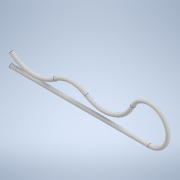
# Autodesk Inventor part: Pin
Saved by Autodesk Inventor 2022 (Build 260153000, 153)
## iProperties
Created: 2022-04-12
Part Number: Pin
Material: Generic
Document SubType Name: Modeling
Designer: Patrick
Density: 1 g/cm^3
Appearance: Default
Author: Patrick
Autodesk Inventor part; units mm, degrees
ref_plane "YZ Plane" through (0, 0, 0) normal (1, 0, 0) x (0, 1, 0)
ref_plane "XZ Plane" through (0, 0, 0) normal (0, 1, 0) x (-1, 0, 0)
ref_plane "XY Plane" through (0, 0, 0) normal (0, 0, 1) x (1, 0, 0)
sketch "Sketch2" plane through (0, 0, 0) normal (0, 0, 1) x (1, 0, 0)
  line L0 (0, 0) -> (75, 0)
  line L1 (149.34, 2.2079) -> (149.4607, 2.2871)
  line L2 (0, 0) -> (0, 4) construction
  arc A0 (75, 0) -> (65.9033, 14.1532) centre (75, 10) ccw
  arc A1 (40.7787, 6.7178) -> (65.9033, 14.1532) centre (50.1063, 21.3655) ccw
  arc A2 (40.7787, 6.7178) -> (23.8868, 5.9248) centre (32.8953, -5.6619) ccw
  arc A3 (0, 6.7617) -> (23.8868, 5.9248) centre (12.4444, 20.6421) ccw
  line L3 (0, 2) -> (24, 2) construction
  line L4 (30, 4) -> (65.9889, 4) construction
  dimension "d3" = 90
  dimension "d4" = 75
  dimension "d6" = 2
  dimension "d9" = 10
  dimension "d10" = 4
  constraints: 10 end point, 8 point on circle, 6 tangent, 4 centre point, 3 horizontal, 1 midpoint
  measures "d3" angle of L0 L2
  measures "d4" distance of L0.start L0.end
  measures "d6" distance between parallel lines of L3 L0
  measures "d9" distance of L0.end A0.centre
  measures "d10" distance between parallel lines of L0 L4
sketch "Sketch3" plane through (0, 0, 0) normal (1, 0, 0) x (0, 1, 0)
  circle A0 centre (0, 0) radius 1
  dimension "d2" = 2
  constraints: 1 centre point, 1 coincident
  measures "d2" diameter of A0
sweep "Sweep1" add profiles "Sketch3" path "Sketch2" path curves L0 A0 A1 A2 A3
body "Solid1"
